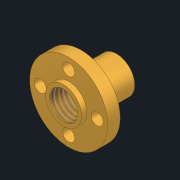
# Autodesk Inventor part: lead-screw-nut
Saved by Autodesk Inventor 2022 (Build 260153000, 153)
## iProperties
Created: 2021-10-11
Part Number: lead-screw-nut
Material: 真鍮、ソフト イエロー
Document SubType Name: Modeling
Designer: Yuta Kage
Density: 8.47 g/cm^3
Appearance: 真鍮 - サテン
Author: Yuta Kage
Autodesk Inventor part; units mm, degrees
ref_plane "YZ Plane" through (0, 0, 0) normal (1, 0, 0) x (0, 1, 0)
ref_plane "XZ Plane" through (0, 0, 0) normal (0, 1, 0) x (-1, 0, 0)
ref_plane "XY Plane" through (0, 0, 0) normal (0, 0, 1) x (1, 0, 0)
sketch "スケッチ1" plane through (0, 0, 0) normal (1, 0, 0) x (0, 1, 0)
  line L0 (0, 0) -> (5.1, 0)
  line L1 (5.1, 0) -> (5.1, -1.5)
  line L2 (5.1, -1.5) -> (11, -1.5)
  line L3 (11, -1.5) -> (11, -5)
  line L4 (11, -5) -> (5.1, -5)
  line L5 (5.1, -5) -> (5.1, -15)
  line L6 (5.1, -15) -> (4, -15)
  line L7 (4, -15) -> (4, 0)
  line L8 (0, -18) -> (0, 3) projected
  dimension "d0" = 4
  dimension "d1" = 1.5
  dimension "d2" = 3.5
  dimension "d3" = 10
  dimension "d4" = 11
  dimension "d5" = 5.1
  constraints: 16 end point, 6 perpendicular, 3 point on line, 1 horizontal
  measures "d0" distance from line of L0.start L7
  measures "d1" distance of L0.end L1.end
  measures "d2" distance of L2.end L3.end
  measures "d3" distance of L4.end L5.end
  measures "d4" distance from line of L3 L0.start
  measures "d5" distance from line of L0.start L1
revolve "回転1" add sketch "スケッチ1" angle 360 about axis through (0, 0, -10) along (0, 0, 1)
sketch "スケッチ2" plane through (0, 0, -1.5) normal (0, 0, 1) x (1, 0, 0)
  circle A0 centre (0, 0) radius 8
  point P0 (0, 8)
  point P1 (-8, 0)
  point P2 (0, -8)
  point P3 (8, 0)
  dimension "d7" = 16
  dimension "d10" = 360
  constraints: 1 coincident, 1 vertical alignment, 7 other
hole "穴1" at (0, 8, -1.5) at (-8, 0, -1.5) at (0, -8, -1.5) at (8, 0, -1.5) direction (0, 0, -1) diameter 3.4 end through all clearance for "Socket Head Cap Screw" size "M3" standard "Ansi Metric M Profile"
thread "ねじ1" size "M8x1.25" class "6H" standard "ANSI Metric M Profile" full length
